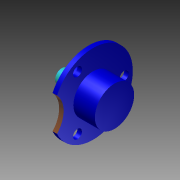
# Autodesk Inventor part: Släpring
Saved by Autodesk Inventor 2012 SP1 (Build 160190100, 190)
## iProperties
Created: 2014-02-18
Part Number: Släpring
Material: Default
Document SubType Name: Modeling
Designer: Pinkponk
Density: 1 g/cm^3
Author: Pinkponk
Autodesk Inventor part; units mm, degrees
ref_plane "YZ Plane" through (0, 0, 0) normal (1, 0, 0) x (0, 1, 0)
ref_plane "XZ Plane" through (0, 0, 0) normal (0, 1, 0) x (-1, 0, 0)
ref_plane "XY Plane" through (0, 0, 0) normal (0, 0, 1) x (1, 0, 0)
sketch "Sketch1" plane through (0, 0, 0) normal (0, 0, 1) x (1, 0, 0)
  line L0 (0, 0) -> (0, 3.8)
  line L1 (0, 3.8) -> (0, 3.8)
  line L2 (0, 3.8) -> (0, 11)
  line L3 (0, 11) -> (5, 11)
  line L4 (5, 11) -> (5, 22.25)
  line L5 (5, 22.25) -> (7.5, 22.25)
  line L6 (7.5, 22.25) -> (7.5, 11)
  line L7 (7.5, 11) -> (19.5, 11)
  line L8 (19.5, 11) -> (19.5, 0)
  line L9 (19.5, 0) -> (0, 0)
  line L10 (0, 0) -> (41.6069, 0)
  dimension "d0" = 7.6
  dimension "d1" = 22
  dimension "d2" = 44.5
  dimension "d3" = 0
  dimension "d4" = 5
  dimension "d5" = 12
  dimension "d6" = 2.5
  constraints: 22 end point, 6 parallel, 2 collinear, 1 horizontal, 1 horizontal alignment, 1 perpendicular, 1 vertical
  measures "d0" diameter of L1 L10
  measures "d1" diameter of L3 L10
  measures "d2" diameter of L5 L10
  measures "d3" distance of L0.end L1.end
  measures "d4" distance of L2.end L3.end
  measures "d5" distance of L6.end L7.end
  measures "d6" distance between parallel lines of L4 L6
revolve "Revolution1" add sketch "Sketch1" angle 360 about axis through (0, 0, 0) along (1, 0, 0)
sketch "Sketch2" plane through (0, 0, 0) normal (-1, 0, 0) x (0, 0, 1)
  circle A0 centre (0, 0) radius 11 projected
  circle A1 centre (0, 0) radius 3.8
  dimension "d8" = 7.6
  constraints: 1 centre point, 1 coincident
  measures "d8" diameter of A1
extrude "Extrusion1" add sketch "Sketch2" along normal blind 10 contours A1
sketch "Sketch3" plane through (7.5, 0, 0) normal (1, 0, 0) x (0, 0, -1)
  circle A0 centre (0, 0) radius 22.25 projected
  circle A1 centre (0, 17.45) radius 2.5
  circle A2 centre (15.1121, -8.725) radius 2.5
  circle A3 centre (-15.1121, -8.725) radius 2.5
  line L0 (0, 0) -> (0, 17.45) construction
  line L1 (0, 0) -> (15.1121, -8.725) construction
  line L2 (0, 0) -> (-15.1121, -8.725) construction
  dimension "d11" = 5
  dimension "d12" = 17.45
  dimension "d13" = 17.45
  dimension "d14" = 17.45
  dimension "d15" = 5
  dimension "d16" = 5
  dimension "d17" = 120
  dimension "d18" = 120
  constraints: 6 end point, 3 centre point, 1 vertical
  measures "d11" diameter of A1
  measures "d12" distance of L0.start L0.end
  measures "d13" distance of L0.start L1.end
  measures "d14" distance of L0.start L2.end
  measures "d15" diameter of A2
  measures "d16" diameter of A3
  measures "d17" angle of L0 L2
  measures "d18" angle of L1 L0
extrude "Extrusion2" cut sketch "Sketch3" against normal through all contours A1 | A2 | A3
sketch "Sketch4" plane through (7.5, 0, 0) normal (1, 0, 0) x (0, 0, -1)
  circle A0 centre (0, 0) radius 11 projected
  circle A1 centre (0, 0) radius 22.25 projected
  arc A2 (9.2992, -20.2135) -> (-9.2992, -20.2135) centre (0, -30) ccw
  dimension "d21" = 13.5
  dimension "d22" = 30
  constraints: 4 point on circle, 1 centre point, 1 vertical alignment
  measures "d21" radius of A2
  measures "d22" distance of A0.centre A2.centre
extrude "Extrusion3" cut sketch "Sketch4" against normal through all contours A2 A1 picked at (-2.0741, -20.1881)
body "Solid1"
